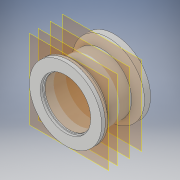
# Autodesk Inventor part: KF50tube_v1
Saved by Autodesk Inventor 2018 (Build 220112000, 112)
## iProperties
Created: 2017-06-29
Part Number: KF50tube_v1
Material: Generic
Document SubType Name: Modeling
Designer: boss
Density: 1 g/cm^3
Appearance: Default
Author: boss
Autodesk Inventor part; units mm, degrees
ref_plane "YZ Plane" through (0, 0, 0) normal (1, 0, 0) x (0, 1, 0)
ref_plane "XZ Plane" through (0, 0, 0) normal (0, 1, 0) x (-1, 0, 0)
sketch "Sketch1" plane through (0, 0, 0) normal (0, 0, 1) x (1, 0, 0)
  circle A0 centre (0, 0) radius 37.465
  dimension "d0" = 74.93
  constraints: 1 centre point, 1 coincident
  measures "d0" diameter of A0
extrude "Extrusion1" add sketch "Sketch1" along normal blind 50.8
sketch "Sketch3" plane through (0, 0, 50.8) normal (0, 0, 1) x (1, 0, 0)
  circle A0 centre (0, 0) radius 26.162
  dimension "d6" = 52.324
  constraints: 1 centre point, 1 coincident
  measures "d6" diameter of A0
extrude "Extrusion3" cut sketch "Sketch3" against normal blind 2.54
sketch "Sketch4" plane through (0, 0, 0) normal (0, 0, -1) x (-1, 0, 0)
  circle A0 centre (0, 0) radius 26.162
  dimension "d9" = 52.324
  constraints: 1 centre point, 1 coincident
  measures "d9" diameter of A0
extrude "Extrusion4" cut sketch "Sketch4" against normal blind 2.54
ref_plane "Work Plane1" through (0, 0, 25.4) normal (0, 0, 1) x (1, 0, 0)
sketch "Sketch5" plane through (0, 0, 25.4) normal (0, 0, 1) x (1, 0, 0)
  circle A0 centre (0, 0) radius 30.48
  circle A1 centre (0, 0) radius 37.465
  dimension "d13" = 60.96
  constraints: 2 centre point, 2 coincident
  measures "d13" diameter of A0
extrude "Extrusion5" cut sketch "Sketch5" along normal mid plane 38.1
ref_plane "Work Plane2" through (0, 0, 38.1) normal (0, 0, 1) x (1, 0, 0)
sketch "Sketch6" plane through (0, 0, 38.1) normal (0, 0, 1) x (1, 0, 0)
  circle A0 centre (0, 0) radius 30.48
  dimension "d17" = 60.96
  constraints: 1 centre point, 1 coincident
  measures "d17" diameter of A0
loft "Loft1" add profiles "Sketch6" section 1 edges at (-37.465, 0, 44.45)
ref_plane "Work Plane3" through (0, 0, 12.7) normal (0, 0, 1) x (1, 0, 0)
sketch "Sketch7" plane through (0, 0, 12.7) normal (0, 0, 1) x (1, 0, 0)
  circle A0 centre (0, 0) radius 30.48
  dimension "d31" = 60.96
  constraints: 1 centre point, 1 coincident
  measures "d31" diameter of A0
loft "Loft3" add profiles "Sketch7" section 1 edges at (-37.465, 0, 6.35)
sketch "Sketch2" plane through (0, 0, 50.8) normal (0, 0, 1) x (1, 0, 0)
  circle A0 centre (0, 0) radius 25.019
  dimension "d3" = 50.038
  constraints: 1 centre point, 1 coincident
  measures "d3" diameter of A0
extrude "Extrusion2" cut sketch "Sketch2" against normal blind 50.8
ref_plane "Work Plane4" through (0, 0, 46.99) normal (0, 0, 1) x (1, 0, 0)
split body "Split2" result two bodies by plane through (0, 0, 46.99) normal (0, 0, 1) first body at (33.0032, 2.7789, 47.49)
body "Solid4"
body "Solid5"
